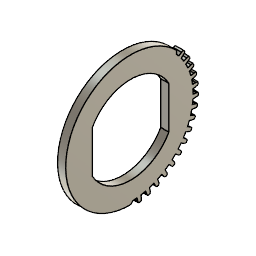
Double-Roller Barrel Throttle_ (Autodesk Fusion 360 archive; units mm, degrees)
design "Gear"
Autodesk Fusion 360 part; units mm, degrees
sketch "Sketch1" plane through (0, 0, 0) normal (1, 0, 0) x (0, 1, 0)
  line L0 (-14, 7.746) -> (-14, -7.746)
  line L1 (14, -7.746) -> (14, 7.746)
  line L2 (0, 0) -> (0, 30.2965) construction
  arc A0 (-14, -7.746) -> (14, -7.746) centre (0, 0) ccw
  arc A1 (14, 7.746) -> (-14, 7.746) centre (0, 0) ccw
  line L3 (16.8429, 16.8154) -> (16.8429, 15.5154)
  line L4 (0.0194, -23.8) -> (0.9387, -22.8808)
  arc A2 (16.8429, 16.8154) -> (0.0194, -23.8) centre (0, 0) ccw
  arc A3 (0.9387, -22.8808) -> (16.8429, 15.5154) centre (0, 0) ccw
  dimension "d1" = 47.6
  dimension "d2" = 32
  dimension "d3" = 28
  dimension "d4" = 45.8
  dimension "d5" = 135
  dimension "d6" = 1.3
  dimension "d7" = 1.3
  constraint coincident L2.start A0.centre
  constraint concentric A0 A2
  constraint vertical L0
  constraint coincident L1.end A0
  constraint parallel L0 L1
  constraint parallel L1 L2
  constraint symmetric L0 L1 L2
  constraint concentric A0 A1
  constraint vertical L3
  measures "d1" diameter of A2
  measures "d2" diameter of A0
  measures "d3" distance of L0 L1
  measures "d4" diameter of A3
  measures "d5" angle of L3 L4
  measures "d6" distance of L4.start L4.end
  measures "d7" distance of L3.start L3.end
extrude "Extrude1" add sketch "Sketch1" along normal blind 3
sketch "Sketch2" plane through (3, 0, 0) normal (1, 0, 0) x (0, 1, 0)
  arc A0 (14, 7.746) -> (-14, 7.746) centre (0, 0) ccw
  line L0 (14, 7.746) -> (14, -7.746)
  arc A1 (-14, -7.746) -> (14, -7.746) centre (0, 0) ccw
  line L1 (-14, -7.746) -> (-14, 7.746)
  arc A2 (16.8429, 16.8154) -> (0.0194, -23.8) centre (0, 0) ccw
  line L2 (0.0194, -23.8) -> (0.9387, -22.8808)
  arc A3 (0.9387, -22.8808) -> (16.8429, 15.5154) centre (0, 0) ccw
  line L3 (16.8429, 15.5154) -> (16.8429, 16.8154)
  line L4 (0, 0) -> (32.1047, 24.8771) construction
  line L5 (17.6325, 14.6118) -> (18.628, 15.2818)
  arc A4 (19.3793, 15.5858) -> (18.628, 15.2818) centre (19.7243, 13.653) ccw
  line L6 (19.3793, 15.5858) -> (19.6549, 15.2301)
  line L7 (18.5513, 13.4261) -> (19.4486, 14.2228)
  arc A5 (19.4486, 14.2228) -> (19.9306, 14.8744) centre (18.1451, 15.691) ccw
  line L8 (19.9306, 14.8744) -> (19.6549, 15.2301)
  dimension "d10" = 1.2
  dimension "d11" = 1.2
  dimension "d12" = 2
  dimension "d13" = 0.45
  dimension "d14" = 0.75
  constraint coincident A0.centre A1.centre
  constraint coincident A3 L5.start
  constraint tangent L5 A4
  constraint coincident L4 L6.end
  constraint perpendicular L4 L6
  constraint symmetric L4 L5.start L7.start
  constraint symmetric L4 L5.end L7.end
  constraint symmetric L4 A4.start A5.end
  constraint symmetric L4 A4 A5
  constraint symmetric L4 L6.end L8.end
  measures "d10" distance of A3.end L5.start
  measures "d11" distance of L5.start L5.end
  measures "d12" distance of L5.start A4.start
  measures "d13" distance of L4 A4.start
  measures "d14" distance of L4 L5.start
extrude "Extrude2" add sketch "Sketch2" against normal blind 3 contours A3 L5 A4 L6 L7 A5 L8
pattern_circular "C-Pattern1" count 16 over 120 about axis through (0, 0, 0) along (-1, 0, 0) of "Extrude2"

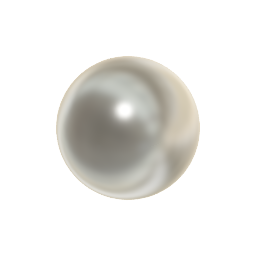
design "Bearing Assembly Ball"
Autodesk Fusion 360 part; units mm, degrees
sketch "Sketch1" plane through (0, 0, 0) normal (0, 1, 0) x (1, 0, 0)
  arc A0 (0, -3) -> (0, 3) centre (0, 0) ccw
  line L0 (0, -3) -> (0, 3)
  dimension "d1" = 3
  constraint coincident A0.centre origin
  constraint vertical L0
  measures "d1" radius of A0
revolve "Revolve1" add sketch "Sketch1" angle 360 about axis through (0, 0, 3) along (0, 0, -1)

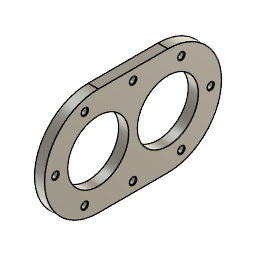
design "Side Plate"
Autodesk Fusion 360 part; units mm, degrees
sketch "Sketch1" plane through (0, 0, 0) normal (1, 0, 0) x (0, 1, 0)
  line L0 (24, 37) -> (-24, 37)
  arc A0 (-24, 37) -> (-24, -37) centre (-24, 0) ccw
  line L1 (-24, -37) -> (24, -37)
  arc A1 (24, -37) -> (24, 37) centre (24, 0) ccw
  line L2 (24, 0) -> (-24, 0) construction
  circle A2 centre (-24, 0) radius 21
  circle A3 centre (24, 0) radius 21
  dimension "d1" = 48
  dimension "d2" = 37
  dimension "d3" = 42
  dimension "d4" = 42
  constraint tangent L0 A0
  constraint tangent A0 L1
  constraint parallel L0 L1
  constraint tangent L1 A1
  constraint tangent L0 A1
  constraint horizontal L2
  constraint midpoint L2 origin
  constraint concentric A0 A2
  constraint concentric A1 A3
  measures "d1" distance of A1.centre A0.centre
  measures "d2" radius of A0
  measures "d3" diameter of A2
  measures "d4" diameter of A3
extrude "Extrude1" add sketch "Sketch1" along normal blind 7
sketch "Sketch2" plane through (7, 0, 0) normal (1, 0, 0) x (0, 1, 0)
  circle A0 centre (-24, 0) radius 21
  circle A1 centre (24, 0) radius 21
  arc A2 (24, -37) -> (24, 37) centre (24, 0) ccw
  line L0 (24, 37) -> (-24, 37)
  arc A3 (-24, 37) -> (-24, -37) centre (-24, 0) ccw
  line L1 (-24, -37) -> (24, -37)
  circle A4 centre (-24, 0) radius 29.5 construction
  line L2 (0, 0) -> (0, 48.4021) construction
  point P0 (0, 30)
  point P1 (-33.2871, 28)
  point P2 (-53.5, 0)
  point P3 (-33.2871, -28)
  point P4 (0, -30)
  point P5 (33.2871, 28)
  point P6 (53.5, 0)
  point P7 (33.2871, -28)
  dimension "d7" = 59
  dimension "d8" = 28
  dimension "d9" = 30
  dimension "d10" = 30
  constraint concentric A0 A4
  constraint coincident L2.start origin
  constraint vertical L2
  constraint coincident L2 P0
  constraint coincident A4 P1
  constraint coincident A4 P2
  constraint coincident A4 P3
  constraint vertical L2.start P4
  constraint horizontal A0.centre P2
  constraint vertical P1 P3
  constraint symmetric L2 P1 P5
  constraint symmetric L2 P2 P6
  constraint symmetric L2 P3 P7
  measures "d7" diameter of A4
  measures "d8" vertical distance of A0.centre P1
  measures "d9" distance of L2.start P0
  measures "d10" distance of L2.start P4
hole "Hole1" at (7, -33.2871, 28) at (7, -53.5, 0) at (7, -33.2871, -28) at (7, 0, -30) at (7, 33.2871, -28) at (7, 53.5, 0) at (7, 33.2871, 28) at (7, 0, 30) direction (-1, 0, 0) diameter 4.2 end through all countersink diameter 5 countersink angle 90

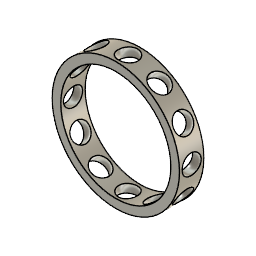
design "Bearing Assembly Cage"
Autodesk Fusion 360 part; units mm, degrees
sketch "Sketch1" plane through (0, 0, 0) normal (0, 1, 0) x (1, 0, 0)
  circle A0 centre (0, 0) radius 18.25
  circle A1 centre (0, 0) radius 15.75
  dimension "d1" = 36.5
  dimension "d2" = 31.5
  constraint coincident A0.centre A1.centre
  constraint concentric A0 A1
  measures "d1" diameter of A0
  measures "d2" diameter of A1
extrude "Extrude1" add sketch "Sketch1" along normal mid plane 7
sketch "Sketch3" plane through (0, 0, 0) normal (0, 1, 0) x (1, 0, 0)
  line L0 (0, 0) -> (0, -29.5716) construction
  arc A0 (0, -14) -> (0, -20) centre (0, -17) ccw
  line L1 (0, -20) -> (0, -14)
  dimension "d5" = 3
  dimension "d6" = 17
  constraint coincident L0.start origin
  constraint vertical L0
  constraint coincident L0 A0.start
  constraint coincident L0 A0.end
  constraint coincident L0 A0.centre
  measures "d5" radius of A0
  measures "d6" distance of L0.start A0.centre
revolve "Revolve1" cut sketch "Sketch3" angle 360 about axis through (0, 0, 0) along (0, 0, 1)
pattern_circular "C-Pattern1" count 12 over 360 about axis through (0, -3.5, 0) along (0, 1, 0) of "Revolve1"

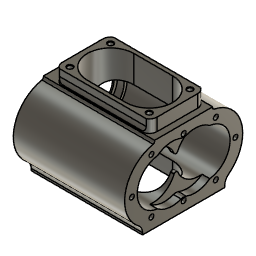
design "Body"
Autodesk Fusion 360 part; units mm, degrees
sketch "Sketch1" plane through (0, 0, 0) normal (1, 0, 0) x (0, 1, 0)
  circle A0 centre (-24, 0) radius 17.5
  arc A1 (-42.5, -37.3731) -> (-46.4362, -29.4214) centre (-52.5, -37.3731) ccw
  arc A2 (-31.4242, 36.2475) -> (-46.4362, -29.4214) centre (-24, 0) ccw
  arc A3 (-31.4242, 36.2475) -> (-30, 39.0239) centre (-31.8255, 38.2068) ccw
  line L0 (-30, 39.0239) -> (0, 39.0239)
  line L1 (0, 39.0239) -> (0, 0) construction
  line L2 (-42.5, -37.3731) -> (-42.5, -39.4214)
  line L3 (-42.5, -39.4214) -> (0, -39.4214)
  line L4 (0, 0) -> (0, -39.4214)
  line L5 (30, 39.0239) -> (0, 39.0239)
  arc A4 (30, 39.0239) -> (31.4242, 36.2475) centre (31.8255, 38.2068) ccw
  arc A5 (46.4362, -29.4214) -> (31.4242, 36.2475) centre (24, 0) ccw
  arc A6 (46.4362, -29.4214) -> (42.5, -37.3731) centre (52.5, -37.3731) ccw
  line L6 (42.5, -37.3731) -> (42.5, -39.4214)
  line L7 (42.5, -39.4214) -> (0, -39.4214)
  line L8 (0, 0) -> (0, -39.4214)
  circle A7 centre (24, 0) radius 17.5
  dimension "d1" = 35
  dimension "d2" = 24
  dimension "d3" = 2
  dimension "d4" = 37
  dimension "d5" = 10
  dimension "d6" = 10
  dimension "d7" = 42.5
  dimension "d8" = 30
  constraint horizontal L1.end A0.centre
  constraint tangent A1 A2
  constraint tangent A2 A3
  constraint horizontal L0
  constraint coincident L1.end L4.start
  constraint concentric A0 A2
  constraint vertical L2
  constraint perpendicular L2 L3
  constraint tangent A1 L2
  constraint vertical L4
  constraint vertical L1
  constraint symmetric A0 L1 A7
  constraint symmetric A1.start L1 A6.end
  constraint symmetric A1.end L1 A5.start
  constraint symmetric A1 L1 A6
  constraint symmetric A2.start L1 A4.end
  constraint symmetric A2 L1 A5
  constraint symmetric A3.end L1 L5.start
  constraint symmetric A3 L1 A4
  constraint symmetric L0.end L1 L5.end
  constraint symmetric L4.start L1 L8.start
  constraint symmetric L1 L2.end L6.end
  constraint symmetric L1 L3.end L4.end
  measures "d1" diameter of A0
  measures "d2" distance of L1.end A0.centre
  measures "d3" radius of A3
  measures "d4" radius of A2
  measures "d5" radius of A1
  measures "d6" vertical distance of A1.end L2.end
  measures "d7" distance of L2.end L3.end
  measures "d8" distance of A3.end L0.end
extrude "Extrude1" add sketch "Sketch1" along normal blind 115
sketch "Sketch2" plane through (115, 0, 0) normal (1, 0, 0) x (0, 1, 0)
  circle A0 centre (-24, 0) radius 17.5
  circle A1 centre (24, 0) radius 17.5
  arc A2 (46.4362, -29.4214) -> (31.4242, 36.2475) centre (24, 0) ccw
  arc A3 (30, 39.0239) -> (31.4242, 36.2475) centre (31.8255, 38.2068) ccw
  line L0 (30, 39.0239) -> (-30, 39.0239)
  arc A4 (-31.4242, 36.2475) -> (-30, 39.0239) centre (-31.8255, 38.2068) ccw
  arc A5 (-31.4242, 36.2475) -> (-46.4362, -29.4214) centre (-24, 0) ccw
  arc A6 (-42.5, -37.3731) -> (-46.4362, -29.4214) centre (-52.5, -37.3731) ccw
  line L1 (-42.5, -37.3731) -> (-42.5, -39.4214)
  line L2 (-42.5, -39.4214) -> (42.5, -39.4214)
  line L3 (42.5, -39.4214) -> (42.5, -37.3731)
  arc A7 (46.4362, -29.4214) -> (42.5, -37.3731) centre (52.5, -37.3731) ccw
  arc A8 (-1.8449, 9.2279) -> (1.8462, 9.2308) centre (0, 10) ccw
  arc A9 (1.8462, -9.2308) -> (-1.8461, -9.2308) centre (0, -10) ccw
  arc A10 (-1.8449, 9.2279) -> (-1.8461, -9.2308) centre (-24, 0) ccw
  arc A11 (1.8462, -9.2308) -> (1.8462, 9.2308) centre (24, 0) ccw
  dimension "d11" = 48
  dimension "d12" = 48
  dimension "d13" = 20
  dimension "d14" = 2
  dimension "d15" = 2
  constraint concentric A0 A10
  constraint concentric A1 A11
  constraint tangent A8 A11
  constraint tangent A9 A11
  measures "d11" diameter of A10
  measures "d12" diameter of A11
  measures "d13" vertical distance of A8.centre A9.centre
  measures "d14" radius of A9
  measures "d15" radius of A8
extrude "Extrude2" cut sketch "Sketch2" against normal blind 106.5 contours A8 A9 A10 A11
sketch "Sketch3" plane through (115, 0, 0) normal (1, 0, 0) x (0, 1, 0)
  arc A0 (1.8462, -9.2308) -> (-1.8461, -9.2308) centre (0, -10) ccw
  arc A1 (-1.8449, 9.2279) -> (-1.8461, -9.2308) centre (-24, 0) ccw
  arc A2 (-1.8449, 9.2279) -> (1.8462, 9.2308) centre (0, 10) ccw
  arc A3 (1.8462, -9.2308) -> (1.8462, 9.2308) centre (24, 0) ccw
  arc A4 (46.4362, -29.4214) -> (31.4242, 36.2475) centre (24, 0) ccw
  arc A5 (30, 39.0239) -> (31.4242, 36.2475) centre (31.8255, 38.2068) ccw
  line L0 (30, 39.0239) -> (-30, 39.0239)
  arc A6 (-31.4242, 36.2475) -> (-30, 39.0239) centre (-31.8255, 38.2068) ccw
  arc A7 (-31.4242, 36.2475) -> (-46.4362, -29.4214) centre (-24, 0) ccw
  arc A8 (-42.5, -37.3731) -> (-46.4362, -29.4214) centre (-52.5, -37.3731) ccw
  line L1 (-42.5, -37.3731) -> (-42.5, -39.4214)
  line L2 (-42.5, -39.4214) -> (42.5, -39.4214)
  line L3 (42.5, -39.4214) -> (42.5, -37.3731)
  arc A9 (46.4362, -29.4214) -> (42.5, -37.3731) centre (52.5, -37.3731) ccw
  line L4 (0, 0) -> (0, 67.4352) construction
  arc A10 (-2.5795, 27.2102) -> (-27, 23.8118) centre (-11.792, 3.9695) ccw
  arc A11 (-2.5795, 27.2102) -> (2.5795, 27.2102) centre (0, 33.7176) ccw
  arc A12 (27, 23.8118) -> (2.5795, 27.2102) centre (11.792, 3.9695) ccw
  dimension "d18" = 7
  dimension "d19" = 25
  dimension "d20" = 54
  constraint coincident L4.start origin
  constraint perpendicular L0 L4
  constraint coincident A1 A10.end
  constraint tangent A10 A11
  constraint tangent A11 A12
  constraint coincident A3 A12.start
  constraint equal A10 A12
  constraint symmetric L4 A10 A12
  constraint midpoint L4 A11.centre
  measures "d18" radius of A11
  measures "d19" radius of A10
  measures "d20" distance of A10.end A12.start
extrude "Extrude3" cut sketch "Sketch3" against normal blind 8 contours A1 A2 A3 A10 A11 A12
sketch "Sketch4" plane through (8.5, 0, 0) normal (1, 0, 0) x (0, 1, 0)
  circle A0 centre (-24, 0) radius 17.5
  circle A1 centre (24, 0) radius 17.5
  arc A2 (-1.8449, 9.2279) -> (-1.8461, -9.2308) centre (-24, 0) ccw
  arc A3 (1.8462, -9.2308) -> (-1.8461, -9.2308) centre (0, -10) ccw
  arc A4 (1.8462, -9.2308) -> (1.8462, 9.2308) centre (24, 0) ccw
  arc A5 (-1.8449, 9.2279) -> (1.8462, 9.2308) centre (0, 10) ccw
  circle A6 centre (-24, 0) radius 21
  circle A7 centre (24, 0) radius 21
  dimension "d23" = 42
  dimension "d24" = 42
  constraint concentric A0 A6
  constraint concentric A1 A7
  measures "d23" diameter of A6
  measures "d24" diameter of A7
extrude "Extrude4" cut sketch "Sketch4" against normal blind 7 contours A6 | A7
sketch "Sketch5" plane through (0, 0, 39.0239) normal (0, 0, 1) x (-1, 0, 0)
  line L0 (0, -30) -> (0, 30)
  line L1 (0, 30) -> (-115, 30)
  line L2 (-115, 30) -> (-115, -30)
  line L3 (-115, -30) -> (0, -30)
  line L4 (-10.5, -29) -> (-108.5, -29)
  line L5 (-108.5, -29) -> (-108.5, 29)
  line L6 (-108.5, 29) -> (-10.5, 29)
  line L7 (-10.5, 29) -> (-10.5, -29)
  line L8 (-10.5, -29) -> (-108.5, 29) construction
  line L9 (-108.5, -29) -> (-10.5, 29) construction
  point P0 (-59.5, 0)
  dimension "d27" = 10.5
  dimension "d28" = 58
  dimension "d29" = 98
  constraint horizontal L4
  constraint perpendicular L4 L5
  constraint parallel L4 L6
  constraint parallel L5 L7
  constraint coincident L8 P0
  constraint coincident L9 P0
  constraint midpoint L8 P0
  constraint horizontal origin P0
  measures "d27" distance of L0 L7
  measures "d28" distance of L4.start L6.end
  measures "d29" distance of L5.end L6.end
extrude "Extrude5" add sketch "Sketch5" along normal blind 13 contours L4 L5 L6 L7
fillet "Fillet1" radius 8 4 edges at (108.5, -29, 45.5239) (108.5, 29, 45.5239) (10.5, 29, 45.5239) (10.5, -29, 45.5239)
sketch "Sketch6" plane through (0, 0, 52.0239) normal (0, 0, 1) x (-1, 0, 0)
  arc A0 (-10.5, 21) -> (-18.5, 29) centre (-18.5, 21) ccw
  line L0 (-18.5, 29) -> (-100.5, 29)
  arc A1 (-100.5, 29) -> (-108.5, 21) centre (-100.5, 21) ccw
  line L1 (-108.5, 21) -> (-108.5, -21)
  arc A2 (-108.5, -21) -> (-100.5, -29) centre (-100.5, -21) ccw
  line L2 (-100.5, -29) -> (-18.5, -29)
  arc A3 (-18.5, -29) -> (-10.5, -21) centre (-18.5, -21) ccw
  line L3 (-10.5, -21) -> (-10.5, 21)
  line L4 (-39.5, 24) -> (-79.5, 24)
  arc A4 (-79.5, 24) -> (-79.5, -24) centre (-79.5, 0) ccw
  line L5 (-79.5, -24) -> (-39.5, -24)
  arc A5 (-39.5, -24) -> (-39.5, 24) centre (-39.5, 0) ccw
  line L6 (-39.5, 0) -> (-79.5, 0) construction
  point P0 (-59.5, 0)
  dimension "d34" = 24
  dimension "d35" = 40
  dimension "d36" = 29
  constraint tangent L4 A4
  constraint tangent A4 L5
  constraint parallel L4 L5
  constraint tangent L5 A5
  constraint tangent L4 A5
  constraint perpendicular L3 L6
  constraint midpoint L6 P0
  constraint horizontal origin P0
  measures "d34" radius of A4
  measures "d35" distance of L4.start L4.end
  measures "d36" distance of L1 A4.centre
extrude "Extrude6" cut sketch "Sketch6" against normal blind 100 contours L4 A4 L5 A5
sketch "Sketch7" plane through (108.5, 0, 0) normal (1, 0, 0) x (0, 1, 0)
  line L0 (21, 39.0239) -> (21, 52.0239)
  line L1 (21, 52.0239) -> (-21, 52.0239)
  line L2 (-21, 52.0239) -> (-21, 39.0239)
  line L3 (-21, 39.0239) -> (21, 39.0239)
  line L4 (-28, 52.0239) -> (-28, 45.0239)
  arc A0 (-29, 40.0239) -> (-28, 45.0239) centre (-41, 45.0239) ccw
  line L5 (-29, 52.0239) -> (-21, 52.0239)
  line L6 (-29, 52.0239) -> (-29, 39.0239)
  dimension "d39" = 1
  dimension "d40" = 1
  dimension "d41" = 7
  constraint vertical L4
  constraint tangent L4 A0
  constraint coincident L4.start L5
  constraint coincident A0.start L6
  measures "d39" distance of L4.start L5.start
  measures "d40" distance of A0.start L6.end
  measures "d41" distance of L4.start L4.end
extrude "Extrude7" cut sketch "Sketch7" against normal up to surface (98 mm away) contours L4 A0 L5 L6
mirror "Mirror1" about plane through (0, 0, 0) normal (0, 1, 0) of "Extrude7"
sketch "Sketch8" plane through (0, 0, 52.0239) normal (0, 0, 1) x (-1, 0, 0)
  line L0 (-104.373, -28) -> (-14.627, -28)
  arc A0 (-14.627, -28) -> (-10.5, -21) centre (-18.5, -21) ccw
  line L1 (-10.5, -21) -> (-10.5, 21)
  arc A1 (-10.5, 21) -> (-14.627, 28) centre (-18.5, 21) ccw
  line L2 (-14.627, 28) -> (-104.373, 28)
  arc A2 (-104.373, 28) -> (-108.5, 21) centre (-100.5, 21) ccw
  line L3 (-108.5, 21) -> (-108.5, -21)
  arc A3 (-108.5, -21) -> (-104.373, -28) centre (-100.5, -21) ccw
  line L4 (-79.5, 24) -> (-39.5, 24)
  arc A4 (-39.5, -24) -> (-39.5, 24) centre (-39.5, 0) ccw
  line L5 (-39.5, -24) -> (-79.5, -24)
  arc A5 (-79.5, 24) -> (-79.5, -24) centre (-79.5, 0) ccw
  circle A6 centre (-100.5, 21) radius 3
  circle A7 centre (-100.5, -21) radius 3
  circle A8 centre (-18.5, -21) radius 3
  circle A9 centre (-18.5, 21) radius 3
  dimension "d46" = 6
  dimension "d47" = 6
  dimension "d48" = 6
  dimension "d49" = 6
  constraint concentric A2 A6
  constraint concentric A3 A7
  constraint concentric A0 A8
  constraint concentric A1 A9
  measures "d46" diameter of A6
  measures "d47" diameter of A7
  measures "d48" diameter of A8
  measures "d49" diameter of A9
hole "Hole1" at (100.5, 21, 52.0239) at (100.5, -21, 52.0239) at (18.5, -21, 52.0239) at (18.5, 21, 52.0239) direction (0, 0, -1) diameter 5 depth 19 tip angle 180 countersink diameter 6 countersink angle 90
sketch "Sketch9" plane through (115, 0, 0) normal (1, 0, 0) x (0, 1, 0)
  arc A0 (27, 23.8118) -> (2.5795, 27.2102) centre (11.792, 3.9695) ccw
  arc A1 (1.8462, -9.2308) -> (27, 23.8118) centre (24, 0) ccw
  arc A2 (1.8462, -9.2308) -> (-1.8461, -9.2308) centre (0, -10) ccw
  arc A3 (-27, 23.8118) -> (-1.8461, -9.2308) centre (-24, 0) ccw
  arc A4 (-2.5795, 27.2102) -> (-27, 23.8118) centre (-11.792, 3.9695) ccw
  arc A5 (-2.5795, 27.2102) -> (2.5795, 27.2102) centre (0, 33.7176) ccw
  arc A6 (46.4362, -29.4214) -> (31.4242, 36.2475) centre (24, 0) ccw
  arc A7 (30, 39.0239) -> (31.4242, 36.2475) centre (31.8255, 38.2068) ccw
  line L0 (30, 39.0239) -> (-30, 39.0239)
  arc A8 (-31.4242, 36.2475) -> (-30, 39.0239) centre (-31.8255, 38.2068) ccw
  arc A9 (-31.4242, 36.2475) -> (-46.4362, -29.4214) centre (-24, 0) ccw
  arc A10 (-42.5, -37.3731) -> (-46.4362, -29.4214) centre (-52.5, -37.3731) ccw
  line L1 (-42.5, -37.3731) -> (-42.5, -39.4214)
  line L2 (-42.5, -39.4214) -> (42.5, -39.4214)
  line L3 (42.5, -39.4214) -> (42.5, -37.3731)
  arc A11 (46.4362, -29.4214) -> (42.5, -37.3731) centre (52.5, -37.3731) ccw
  circle A12 centre (-24, 0) radius 29.5 construction
  line L4 (0, 0) -> (0, 37.1626) construction
  point P0 (-33.2871, 28)
  point P1 (-53.5, 0)
  point P2 (-33.2871, -28)
  point P3 (0, -30)
  point P4 (0, 30)
  point P5 (33.2871, 28)
  point P6 (53.5, 0)
  point P7 (33.2871, -28)
  dimension "d55" = 59
  dimension "d56" = 28
  dimension "d57" = 30
  dimension "d58" = 30
  constraint concentric A3 A12
  constraint coincident A12 P0
  constraint coincident A12 P1
  constraint coincident A12 P2
  constraint coincident L4.start origin
  constraint vertical L4
  constraint horizontal L4.start P1
  constraint vertical L4.start P4
  constraint vertical P0 P2
  constraint vertical L4.start P3
  constraint symmetric P0 L4 P5
  constraint symmetric P1 L4 P6
  constraint symmetric P2 L4 P7
  measures "d55" diameter of A12
  measures "d56" vertical distance of A3.centre P0
  measures "d57" distance of L4.start P4
  measures "d58" distance of L4.start P3
hole "Hole2" at (115, 0, 30) at (115, -33.2871, 28) at (115, -53.5, 0) at (115, -33.2871, -28) at (115, 0, -30) at (115, 33.2871, -28) at (115, 53.5, 0) at (115, 33.2871, 28) direction (-1, 0, 0) diameter 5 depth 8 tip angle 118
mirror "Mirror2" about plane through (0, 0, 0) normal (0, 0, 1) of "Extrude3"

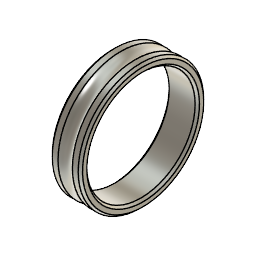
design "Bearing Assembly Inner Ring"
Autodesk Fusion 360 part; units mm, degrees
sketch "Sketch2" plane through (0, 0, 0) normal (0, 1, 0) x (1, 0, 0)
  line L0 (0, 0) -> (0, -17.2519) construction
  line L1 (0, -17.2519) -> (0, 0) construction
  line L2 (0, 0) -> (-10.0877, 0) construction
  line L3 (-1.6583, -14.5) -> (-3.5, -14.5)
  line L4 (-3.5, -14.5) -> (-3.5, -12.5)
  line L5 (-3.5, -12.5) -> (3.5, -12.5)
  line L6 (3.5, -12.5) -> (3.5, -14.5)
  line L7 (3.5, -14.5) -> (1.6583, -14.5)
  arc A0 (1.6583, -14.5) -> (-1.6583, -14.5) centre (0, -17) ccw
  dimension "d7" = 29
  dimension "d8" = 25
  dimension "d9" = 7
  dimension "d10" = 3
  dimension "d12" = 17
  constraint coincident L0.start L1.end
  constraint vertical L0
  constraint perpendicular L1 L2
  constraint perpendicular L3 L4
  constraint perpendicular L4 L5
  constraint perpendicular L5 L6
  constraint perpendicular L4 L7
  constraint symmetric L0 L3 L7
  constraint equal L3 L7
  measures "d9" distance of L4 L6
  measures "d10" radius of A0
  measures "d12" vertical distance of L0.start A0.centre
revolve "Revolve1" add sketch "Sketch2" angle 360 about axis through (1.75, 0, 0) along (1, 0, 0)
chamfer "Chamfer1" distance 0.5 angle 45 4 edges at (-3.5, -5.2434, -13.5187) (3.5, -5.2434, -13.5187) (-3.5, -4.5202, -11.6541) (3.5, -4.5202, -11.6541)

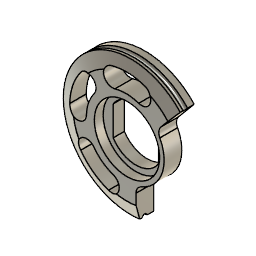
design "Driver Wheel"
Autodesk Fusion 360 part; units mm, degrees
sketch "Sketch1" plane through (0, 0, 0) normal (1, 0, 0) x (0, 1, 0)
  line L0 (2.25, 0) -> (9, 0)
  line L1 (9, 0) -> (9, 13)
  line L2 (9, 13) -> (10, 13)
  line L3 (8, 13.0018) -> (8, 30.0018)
  line L4 (0.1376, 24.0019) -> (0.043, 7.5003)
  line L5 (2.25, 0) -> (0.043, 7.5003)
  line L6 (1.772, 30.0018) -> (0.1376, 24.0019)
  arc A0 (3, 30.0018) -> (5, 30.0018) centre (4, 30.0018) ccw
  line L7 (8, 30.0018) -> (5, 30.0018)
  line L8 (3, 30.0018) -> (1.772, 30.0018)
  line L9 (0.043, 7.5003) -> (0, 0)
  line L10 (0, 0) -> (2.25, 0)
  line L11 (2.25, 0) -> (9, 0)
  line L12 (9, 13) -> (9, 0)
  line L13 (9, 13) -> (8, 13.0018)
  point P0 (0.172, 30.0018)
  dimension "d1" = 9
  dimension "d2" = 13
  dimension "d3" = 17
  dimension "d4" = 1
  dimension "d5" = 2.25
  dimension "d6" = 7.5005
  dimension "d7" = 1.6
  dimension "d8" = 6
  dimension "d9" = 1
  dimension "d10" = 3
  constraint coincident L9.end L10.start
  constraint horizontal L0
  constraint perpendicular L0 L1
  constraint perpendicular L1 L2
  constraint perpendicular L2 L3
  constraint perpendicular L3 L7
  constraint coincident L9.end L0
  constraint coincident L9.end L4
  constraint coincident P0 L7
  constraint coincident P0 L4
  constraint coincident A0.start L7
  constraint collinear L7 L8
  constraint coincident A0.centre L7
  measures "d1" distance of L9.end L0.end
  measures "d2" distance of L0.end L1.end
  measures "d3" distance of L3.start L3.end
  measures "d4" distance of L1.end L3.start
  measures "d5" distance of L9.end L0.start
  measures "d6" distance of L9.end L4.end
  measures "d7" distance of P0 L6.start
  measures "d8" distance of P0 L4.start
  measures "d9" radius of A0
  measures "d10" distance of L3.end A0.end
revolve "Revolve1" add sketch "Sketch1" angle 360 about axis through (0, 2.25, 0) along (0, 1, 0)
sketch "Sketch2" plane through (0, 0, 0) normal (0, 1, 0) x (1, 0, 0)
  arc A0 (-5.3869, -16.5801) -> (5.1945, -16.313) centre (-0.5171, 0.2287) ccw
  arc A1 (-5.3869, -16.5801) -> (-7.6131, -24.2641) centre (-6.5, -20.4221) ccw
  arc A2 (-7.6131, -24.2641) -> (7.8055, -23.8749) centre (-0.5171, 0.2287) ccw
  arc A3 (7.8055, -23.8749) -> (5.1945, -16.313) centre (6.5, -20.094) ccw
  arc A4 (-6.5, -20.4221) -> (6.5, -20.094) centre (-0.5171, 0.2287) ccw construction
  arc A5 (-26.0101, -0.3689) -> (-21.0025, -14.9569) centre (-0.5171, 0.2287) ccw
  arc A6 (-21.0025, -14.9569) -> (-14.5757, -10.1928) centre (-17.7891, -12.5748) ccw
  arc A7 (-18.0123, -0.1814) -> (-14.5757, -10.1928) centre (-0.5171, 0.2287) ccw
  arc A8 (-18.0123, -0.1814) -> (-26.0101, -0.3689) centre (-22.0112, -0.2752) ccw
  arc A9 (-8.7529, 24.3621) -> (-21.1599, 15.1995) centre (-0.5171, 0.2287) ccw
  arc A10 (-21.1599, 15.1995) -> (-14.6837, 10.5028) centre (-17.9218, 12.8512) ccw
  arc A11 (-6.1692, 16.7908) -> (-14.6837, 10.5028) centre (-0.5171, 0.2287) ccw
  arc A12 (-6.1692, 16.7908) -> (-8.7529, 24.3621) centre (-7.461, 20.5765) ccw
  line L0 (0, 0) -> (0, -45.0987) construction
  line L1 (0, 0) -> (49.3466, 0) construction
  circle A13 centre (0, 0) radius 16.5
  line L2 (22, -20.3988) -> (15.0673, -12.1367)
  arc A14 (14.5936, -7.6991) -> (15.0673, -12.1367) centre (18.1315, -9.5655) ccw
  line L3 (4, 29.734) -> (4, 18.8746)
  arc A15 (4, 18.8746) -> (6.439, 15.1917) centre (8, 18.8746) ccw
  circle A16 centre (0, 0) radius 30.0018
  dimension "d12" = 4
  dimension "d13" = 25.5
  dimension "d14" = 6.5
  dimension "d15" = 6.5
  dimension "d17" = -145
  dimension "d18" = 33
  dimension "d19" = 140
  dimension "d20" = 4
  dimension "d21" = 4
  dimension "d22" = 4
  dimension "d23" = 22
  constraint tangent A0 A1
  constraint tangent A1 A2
  constraint tangent A2 A3
  constraint tangent A0 A3
  constraint coincident L0.start L1.start
  constraint vertical L0
  constraint perpendicular L0 L1
  constraint coincident A13 A14.start
  constraint tangent L2 A14
  constraint tangent A13 A14
  constraint vertical L3
  constraint coincident A13 A15.end
  constraint tangent L3 A15
  constraint tangent A13 A15
  constraint coincident L3.start A16
  constraint coincident L2.start A16
  measures "d12" radius of A1
  measures "d13" radius of A2
  measures "d14" horizontal distance of L0.start A1.centre
  measures "d15" horizontal distance of L0.start A3.centre
  measures "d18" diameter of A13
  measures "d19" angle of L2 L3
  measures "d20" radius of A15
  measures "d21" radius of A14
  measures "d22" distance of L0.start L3
  measures "d23" distance of L0 L2.start
extrude "Extrude1" cut sketch "Sketch2" along normal up to surface (8 mm away) contours A0 A1 A2 A3 | A5 A6 A7 A8 | A9 A10 A11 A12 | A13 L2 A14 L3 A15 A16 picked at (8.2829, 20.1154)
sketch "Sketch3" plane through (0, 8, 0) normal (0, 1, 0) x (-1, 0, 0)
  line L0 (-4, -18.8746) -> (-4, -29.734)
  arc A0 (-4, -29.734) -> (-22, 20.3988) centre (0, 0) ccw
  line L1 (-22, 20.3988) -> (-15.0673, 12.1367)
  arc A1 (-14.5936, 7.6991) -> (-15.0673, 12.1367) centre (-18.1315, 9.5655) ccw
  arc A2 (-14.5936, 7.6991) -> (-6.439, -15.1917) centre (0, 0) ccw
  arc A3 (-4, -18.8746) -> (-6.439, -15.1917) centre (-8, -18.8746) ccw
  arc A4 (26.0101, 0.3689) -> (21.0025, 14.9569) centre (0.5171, -0.2287) ccw
  arc A5 (18.0123, 0.1814) -> (26.0101, 0.3689) centre (22.0112, 0.2752) ccw
  arc A6 (18.0123, 0.1814) -> (14.5757, 10.1928) centre (0.5171, -0.2287) ccw
  arc A7 (21.0025, 14.9569) -> (14.5757, 10.1928) centre (17.7891, 12.5748) ccw
  arc A8 (8.7529, -24.3621) -> (21.1599, -15.1995) centre (0.5171, -0.2287) ccw
  arc A9 (6.1692, -16.7908) -> (8.7529, -24.3621) centre (7.461, -20.5765) ccw
  arc A10 (6.1692, -16.7908) -> (14.6837, -10.5028) centre (0.5171, -0.2287) ccw
  arc A11 (21.1599, -15.1995) -> (14.6837, -10.5028) centre (17.9218, -12.8512) ccw
  arc A12 (7.6131, 24.2641) -> (-7.8055, 23.8749) centre (0.5171, -0.2287) ccw
  arc A13 (5.3869, 16.5801) -> (7.6131, 24.2641) centre (6.5, 20.4221) ccw
  arc A14 (5.3869, 16.5801) -> (-5.1945, 16.313) centre (0.5171, -0.2287) ccw
  arc A15 (-7.8055, 23.8749) -> (-5.1945, 16.313) centre (-6.5, 20.094) ccw
  circle A16 centre (0, 0) radius 13.0018
  line L2 (10.05, 6.5572) -> (10.05, -6.5572)
  line L3 (-10.05, 6.5572) -> (-10.05, -6.5572)
  line L4 (0, 0) -> (0, 20.9906) construction
  arc A17 (10.05, 6.5572) -> (-10.05, 6.5572) centre (0, 0) ccw
  arc A18 (-10.05, -6.5572) -> (10.05, -6.5572) centre (0, 0) ccw
  dimension "d26" = 24
  dimension "d27" = 20.1
  constraint coincident A0.centre A2.centre
  constraint vertical L2
  constraint coincident L3.end A17
  constraint parallel L2 L3
  constraint symmetric L2 L3 L4
  constraint concentric A17 A18
  measures "d26" diameter of A17
  measures "d27" distance of L2 L3
extrude "Extrude2" cut sketch "Sketch3" along normal blind -76 and the other way blind -16 contours L2 L3 A17 A18
sketch "Sketch6" plane through (0, 0, 0) normal (0, 1, 0) x (1, 0, 0)
  circle A0 centre (0, 0) radius 14.5
  line L0 (10.05, -6.5573) -> (10.05, 6.5573)
  line L1 (0, 0) -> (0, -5.2001) construction
  line L2 (-10.05, -6.5573) -> (-10.05, 6.5573)
  arc A1 (10.05, -6.5573) -> (10.05, 6.5573) centre (0, 0) ccw
  arc A2 (-10.05, 6.5573) -> (-10.05, -6.5573) centre (0, 0) ccw
  dimension "d36" = 29
  dimension "d37" = 24
  constraint coincident A0.centre L1.start
  constraint vertical L0
  constraint parallel L0 L1
  constraint symmetric L0.start L1 L2.start
  constraint symmetric L0.end L1 L2.end
  constraint concentric A1 A2
  measures "d36" diameter of A0
  measures "d37" diameter of A1
extrude "Extrude4" cut sketch "Sketch6" along normal blind 4 contours A0 | L0 A1 | L2 A2
extrude "Extrude3" [rolled back] along distance 1 taper angle 0

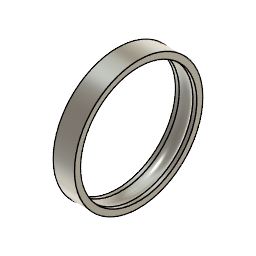
design "Bearing Assembly Outer Ring"
Autodesk Fusion 360 part; units mm, degrees
sketch "Sketch1" plane through (0, 0, 0) normal (0, 1, 0) x (1, 0, 0)
  line L0 (0, 0) -> (-46.3404, 0) construction
  line L1 (-46.3404, 0) -> (0, 0) construction
  line L2 (0, 0) -> (0, -63.877) construction
  line L3 (-2.2361, -19) -> (-3.5, -19)
  line L4 (-3.5, -19) -> (-3.5, -21)
  line L5 (-3.5, -21) -> (3.5, -21)
  line L6 (3.5, -21) -> (3.5, -19)
  line L7 (3.5, -19) -> (2.2361, -19)
  arc A0 (-2.2361, -19) -> (2.2361, -19) centre (0, -17) ccw
  dimension "d1" = 3
  dimension "d2" = 7
  dimension "d3" = 42
  dimension "d4" = 38
  dimension "d5" = 17
  constraint coincident L0.start L1.end
  constraint horizontal L0
  constraint perpendicular L0 L2
  constraint perpendicular L2 L3
  constraint perpendicular L3 L4
  constraint perpendicular L2 L5
  constraint perpendicular L5 L6
  constraint perpendicular L6 L7
  constraint equal L3 L7
  constraint horizontal L3.start L7.end
  measures "d1" radius of A0
  measures "d2" distance of L4.end L5.end
  measures "d5" distance of L0.start A0.centre
revolve "Revolve1" add sketch "Sketch1" angle 360 about axis through (1.75, 0, 0) along (1, 0, 0)
